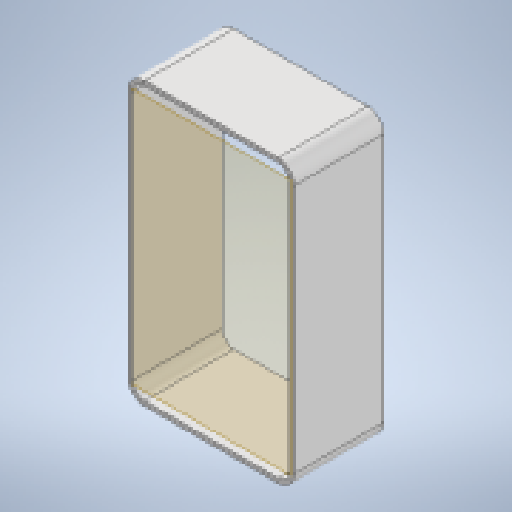
# Autodesk Inventor part: wisecoco-case-body
Saved by Autodesk Inventor 2024 (Build 280153000, 153)
## iProperties
Created: 2024-08-25
Part Number: wisecoco-case-body
Material: Generic
Document SubType Name: Modeling
Designer: Stefano
Density: 1 g/cm^3
Appearance: Default
Author: Stefano
Autodesk Inventor part; units mm, degrees
ref_plane "YZ Plane" through (0, 0, 0) normal (1, 0, 0) x (0, 1, 0)
ref_plane "XZ Plane" through (0, 0, 0) normal (0, 1, 0) x (-1, 0, 0)
ref_plane "XY Plane" through (0, 0, 0) normal (0, 0, 1) x (1, 0, 0)
ref_plane "Work Plane1" through (0, 0, 0) normal (0, 0, 1) x (1, 0, 0)
sketch "Sketch1" plane through (0, 0, 0) normal (0, 0, 1) x (1, 0, 0)
  line L0 (47.5, 99.9) -> (-47.5, 99.9)
  line L1 (-58.9, 88.5) -> (-58.9, -88.5)
  line L2 (-47.5, -99.9) -> (47.5, -99.9)
  line L3 (58.9, -88.5) -> (58.9, 88.5)
  line L4 (58.9, 99.9) -> (-58.9, -99.9) construction
  line L5 (-58.9, 99.9) -> (58.9, -99.9) construction
  arc A0 (58.9, 88.5) -> (47.5, 99.9) centre (47.5, 88.5) ccw
  arc A1 (-47.5, 99.9) -> (-58.9, 88.5) centre (-47.5, 88.5) ccw
  arc A2 (47.5, -99.9) -> (58.9, -88.5) centre (47.5, -88.5) ccw
  arc A3 (-58.9, -88.5) -> (-47.5, -99.9) centre (-47.5, -88.5) ccw
  line L6 (-47.5, 96.9) -> (47.5, 96.9)
  arc A4 (55.9, 88.5) -> (47.5, 96.9) centre (47.5, 88.5) ccw
  line L7 (55.9, 88.5) -> (55.9, -88.5)
  arc A5 (47.5, -96.9) -> (55.9, -88.5) centre (47.5, -88.5) ccw
  line L8 (47.5, -96.9) -> (-47.5, -96.9)
  arc A6 (-55.9, -88.5) -> (-47.5, -96.9) centre (-47.5, -88.5) ccw
  line L9 (-55.9, -88.5) -> (-55.9, 88.5)
  arc A7 (-47.5, 96.9) -> (-55.9, 88.5) centre (-47.5, 88.5) ccw
  point P0 (0, 0)
  dimension "d0" = 199.8
  dimension "d1" = 117.8
  dimension "d2" = 11.4
  dimension "d3" = 3
  constraints: 20 end point, 16 point on circle, 8 centre point, 8 point on line, 8 tangent, 4 parallel, 3 equal radius, 2 midpoint, 2 perpendicular, 1 horizontal, 7 other
  measures "d0" distance between parallel lines of L2 L0
  measures "d1" distance between parallel lines of L1 L3
  measures "d2" radius of A0
  measures "d3" distance between parallel lines of L0 L6
extrude "Extrusion1" add sketch "Sketch1" against normal blind 56.9
ref_plane "Work Plane2" through (0, 0, -6.508) normal (0, 0, -1) x (-1, 0, 0)
sketch "Sketch2" plane through (0, 0, -6.508) normal (0, 0, -1) x (-1, 0, 0)
  arc A0 (-36, 95.8) -> (-24, 95.8) centre (-30, 95.8) ccw construction
  arc A1 (24, 95.8) -> (36, 95.8) centre (30, 95.8) ccw construction
  arc A2 (-24, -95.8) -> (-36, -95.8) centre (-30, -95.8) ccw construction
  arc A3 (36, -95.8) -> (24, -95.8) centre (30, -95.8) ccw construction
  line L0 (47.5, -96.9) -> (-47.5, -96.9) projected
  line L1 (-47.5, 96.9) -> (47.5, 96.9) projected
  circle A4 centre (-30, 95.8) radius 6
  circle A5 centre (30, 95.8) radius 6
  circle A6 centre (-30, 93.8) radius 1.5 construction
  circle A7 centre (30, 93.8) radius 1.5 construction
  circle A8 centre (30, -93.8) radius 1.5 construction
  circle A9 centre (-30, -93.8) radius 1.5 construction
  circle A10 centre (30, -93.8) radius 2
  circle A11 centre (-30, -93.8) radius 2
  circle A12 centre (30, 93.8) radius 2
  circle A13 centre (-30, 93.8) radius 2
  circle A14 centre (30, -95.8) radius 6
  circle A15 centre (-30, -95.8) radius 6
  point P0 (0, 0)
  point P1 (24.1017, 96.9)
  point P2 (35.8983, 96.9)
  point P3 (-35.8983, 96.9)
  point P4 (-24.1017, 96.9)
  point P5 (35.8983, -96.9)
  point P6 (24.1017, -96.9)
  point P7 (-24.1017, -96.9)
  point P8 (-35.8983, -96.9)
  dimension "d6" = 4
  constraints: 8 centre point, 8 coincident, 7 equal radius
  measures "d6" diameter of A10
extrude "Extrusion2" add sketch "Sketch2" along normal blind 3 contours L0 A14 | L0 A15 | L1 A4 | L1 A5 picked at (29.9196, -96.5285) picked at (-30.0804, -96.5285) picked at (-30.0804, 96.5285) picked at (29.9196, 96.5285)
fillet "Fillet1" radius 3.175 8 edges at (24.1017, 96.9, -8.008) (35.8983, 96.9, -8.008) (-24.1017, 96.9, -8.008) (-35.8983, 96.9, -8.008) (-35.8983, -96.9, -8.008) (-24.1017, -96.9, -8.008) (24.1017, -96.9, -8.008) (35.8983, -96.9, -8.008)
sketch "Sketch3" plane through (0, 0, -9.508) normal (0, 0, -1) x (-1, 0, 0)
  circle A0 centre (30, -93.8) radius 2 projected
  circle A1 centre (30, -93.8) radius 3.3
  circle A2 centre (-30, -93.8) radius 2 projected
  circle A3 centre (-30, -93.8) radius 3.3
  circle A4 centre (30, 93.8) radius 2 projected
  circle A5 centre (30, 93.8) radius 3.3
  circle A6 centre (-30, 93.8) radius 2 projected
  circle A7 centre (-30, 93.8) radius 3.3
  line L0 (38.9373, -96.9) -> (21.0627, -96.9) projected
  line L1 (-21.0627, -96.9) -> (-38.9373, -96.9) projected
  line L2 (21.0627, 96.9) -> (38.9373, 96.9) projected
  line L3 (-38.9373, 96.9) -> (-21.0627, 96.9) projected
  point P0 (0, 0)
  point P1 (-31.1314, -96.9)
  point P2 (-28.8686, -96.9)
  point P3 (28.8686, -96.9)
  point P4 (31.1314, -96.9)
  point P5 (-28.8686, 96.9)
  point P6 (-31.1314, 96.9)
  point P7 (31.1314, 96.9)
  point P8 (28.8686, 96.9)
  dimension "d10" = 6.6
  constraints: 4 centre point, 4 coincident, 3 equal radius
  measures "d10" diameter of A1
extrude "Extrusion3" cut sketch "Sketch3" against normal blind 1 contours A1 L0 | A3 L1 | A5 L2 | A7 L3 picked at (29.9196, -96.5285) picked at (-30.0804, -96.5285) picked at (29.9196, 96.5285) picked at (-30.0804, 96.5285)
chamfer "Chamfer1" distance 3 angle 45 8 edges at (-35.0343, -96.9, -9.508) (-24.9657, -96.9, -9.508) (24.9657, -96.9, -9.508) (35.0343, -96.9, -9.508) (-35.0343, 96.9, -9.508) (-24.9657, 96.9, -9.508) (24.9657, 96.9, -9.508) (35.0343, 96.9, -9.508)
ref_plane "Work Plane3" through (-19.1425, -39.31, -52.204) normal (0, 0, -1) x (0, 1, 0)
sketch "Sketch4" plane through (-19.1425, -39.31, -52.204) normal (0, 0, -1) x (0, 1, 0)
  circle A0 centre (9.385, -21.7125) radius 2.25 construction
  circle A1 centre (87.385, -21.7125) radius 2.25 construction
  circle A2 centre (87.385, 63.2875) radius 2.25 construction
  circle A3 centre (9.385, 63.2875) radius 2.25 construction
  circle A4 centre (9.385, -21.7125) radius 5
  circle A5 centre (87.385, -21.7125) radius 5
  circle A6 centre (9.385, 63.2875) radius 5
  circle A7 centre (87.385, 63.2875) radius 5
  line L0 (-49.19, -36.7575) -> (127.81, -36.7575) projected
  line L1 (4.385, -36.7575) -> (4.385, -21.7125)
  line L2 (14.385, -21.7125) -> (14.385, -36.7575)
  line L3 (82.385, -21.7125) -> (82.385, -36.7575)
  line L4 (92.385, -21.7125) -> (92.385, -36.7575)
  line L5 (4.385, 63.2875) -> (4.385, 75.0425)
  line L6 (127.81, 75.0425) -> (-49.19, 75.0425) projected
  line L7 (14.385, 63.2875) -> (14.385, 75.0425)
  line L8 (82.385, 63.2875) -> (82.385, 75.0425)
  line L9 (92.385, 63.2875) -> (92.385, 75.0425)
  circle A8 centre (9.385, -21.7125) radius 1.5
  circle A9 centre (87.385, -21.7125) radius 1.5
  circle A10 centre (9.385, 63.2875) radius 1.5
  circle A11 centre (87.385, 63.2875) radius 1.5
  point P0 (39.31, 19.1425)
  dimension "d16" = 10
  dimension "d17" = 3
  constraints: 16 end point, 8 centre point, 8 coincident, 8 perpendicular, 8 point on circle, 8 point on line, 8 tangent, 6 equal radius
  measures "d16" diameter of A4
  measures "d17" diameter of A8
extrude "Extrusion4" add sketch "Sketch4" against normal blind 4
chamfer "Chamfer2" distance 6 angle 45 4 edges at (-55.9, -29.925, -48.204) (-55.9, 48.075, -48.204) (55.9, 48.075, -48.204) (55.9, -29.925, -48.204)
fillet "Fillet2" radius 2 40 edges at (52.9, -34.925, -45.204) (52.9, -24.925, -45.204) (39.145, -29.925, -48.204) (47.0225, -34.925, -48.204) (47.0225, -24.925, -48.204) (55.9, -34.925, -45.204) (55.9, -34.925, -50.204) (55.9, -29.925, -42.204) (55.9, -24.925, -45.204) (55.9, -24.925, -50.204) (55.9, 43.075, -45.204) (55.9, 43.075, -50.204) (55.9, 48.075, -42.204) (52.9, 43.075, -45.204) (39.145, 48.075, -48.204) (47.0225, 53.075, -48.204) (47.0225, 43.075, -48.204) (52.9, 53.075, -45.204) (55.9, 53.075, -45.204) (55.9, 53.075, -50.204) (-55.9, 43.075, -45.204) (-55.9, 43.075, -50.204) (-55.9, 48.075, -42.204) (-55.9, 53.075, -45.204) (-55.9, 53.075, -50.204) (-52.9, 53.075, -45.204) (-52.9, 43.075, -45.204) (-35.855, 48.075, -48.204) (-45.3775, 43.075, -48.204) (-45.3775, 53.075, -48.204) (-55.9, -34.925, -45.204) (-55.9, -34.925, -50.204) (-55.9, -29.925, -42.204) (-52.9, -24.925, -45.204) (-52.9, -34.925, -45.204) (-35.855, -29.925, -48.204) (-45.3775, -24.925, -48.204) (-45.3775, -34.925, -48.204) (-55.9, -24.925, -45.204) (-55.9, -24.925, -50.204)
ref_plane "Work Plane4" through (0, 0, -53.892) normal (0, 0, 1) x (1, 0, 0)
sketch "Sketch5" plane through (0, 0, -53.892) normal (0, 0, 1) x (1, 0, 0)
  circle A0 centre (47.5, 88.5) radius 2 construction
  circle A1 centre (47.5, -88.5) radius 2 construction
  circle A2 centre (-47.5, -88.5) radius 2 construction
  circle A3 centre (-47.5, 88.5) radius 2 construction
  circle A4 centre (47.5, 88.5) radius 5
  line L0 (47.5, 83.5) -> (55.9, 83.5)
  line L1 (55.9, -88.5) -> (55.9, 88.5) projected
  line L2 (42.5, 88.5) -> (42.5, 96.9)
  line L3 (47.5, 96.9) -> (-47.5, 96.9) projected
  circle A5 centre (47.5, 88.5) radius 1.5
  arc A6 (55.9, 88.5) -> (47.5, 96.9) centre (47.5, 88.5) ccw projected
  point P0 (0, 0)
  dimension "d24" = 10
  dimension "d25" = 3
  constraints: 4 end point, 2 centre point, 2 coincident, 2 perpendicular, 2 point on circle, 2 point on line, 2 tangent
  measures "d24" diameter of A4
  measures "d25" diameter of A5
extrude "Extrusion5" add sketch "Sketch5" along normal blind 4
ref_plane "Work Plane5" through (0, -88.5, 0) normal (-1, 0, 0) x (0, 0, 1)
ref_plane "Work Plane6" through (-47.5, 0, 0) normal (0, -1, 0) x (1, 0, 0)
mirror "Mirror1" about plane through (-47.5, 0, 0) normal (0, -1, 0) of "Extrusion5"
mirror "Mirror2" about plane through (0, -88.5, 0) normal (-1, 0, 0) of "Extrusion5"
mirror "Mirror3" about plane through (-47.5, 0, 0) normal (0, -1, 0) of "Extrusion5", "Mirror2"
chamfer "Chamfer3" distance 2 angle 45 12 edges at (53.4397, 94.4397, -49.892) (55.9, 86, -49.892) (45, 96.9, -49.892) (55.9, -86, -49.892) (53.4397, -94.4397, -49.892) (45, -96.9, -49.892) (-53.4397, 94.4397, -49.892) (-45, 96.9, -49.892) (-55.9, 86, -49.892) (-53.4397, -94.4397, -49.892) (-55.9, -86, -49.892) (-45, -96.9, -49.892)
body "Solid1"
